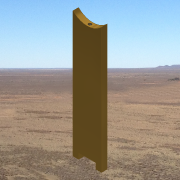
# Autodesk Inventor part: 2f1ar
Saved by Autodesk Inventor 2014 SP1 (Build 180222100, 222)
## iProperties
Company: HERA Project
Created: 2013-12-20
Part Number: 2f1ar
Material: Brass, Soft Yellow
Document SubType Name: Modeling
Designer: Rich Bradley
Mass: 28.2753 g
Surface Area: 26.7824 cm^2
Volume: 3.33829 cm^3
Density: 8.47 g/cm^3
Description: Feed arm pipe rest
Appearance: Brass - Satin
Author: David DeBoer
Title: Dipole Arm Rest
Autodesk Inventor part; units mm, degrees
ref_plane "YZ Plane" through (0, 0, 0) normal (1, 0, 0) x (0, 1, 0)
ref_plane "XZ Plane" through (0, 0, 0) normal (0, 1, 0) x (-1, 0, 0)
sketch "Sketch1" plane through (0, 0, 0) normal (0, 0, 1) x (1, 0, 0)
  line L0 (0, 0) -> (15.875, 0)
  line L1 (15.875, 0) -> (15.875, 77.724)
  line L2 (15.875, 77.724) -> (0, 77.724)
  line L3 (0, 77.724) -> (0, 0)
  dimension "d0" = 77.724
  dimension "d1" = 15.875
  constraints: 8 end point, 2 parallel, 1 horizontal, 1 perpendicular
  measures "d0" distance of L2.end L0.start
  measures "d1" distance of L0.start L0.end
extrude "Extrusion1" add sketch "Sketch1" along normal blind 3.175
sketch "Sketch2" plane through (0, 0, 3.175) normal (0, 0, 1) x (1, 0, 0)
  line L0 (0, 0) -> (15.875, 0) projected
  line L1 (15.875, 77.724) -> (0, 77.724) projected
  line L2 (3.175, 0) -> (12.7, 0)
  line L3 (12.7, 0) -> (12.7, 3.175)
  line L4 (12.7, 3.175) -> (3.175, 3.175)
  line L5 (3.175, 3.175) -> (3.175, 0)
  line L6 (7.9375, 3.175) -> (7.9375, 0) construction
  line L7 (7.9375, 77.724) -> (7.9375, 0) construction
  dimension "d4" = 9.525
  dimension "d6" = 3.175
  constraints: 12 end point, 4 midpoint, 2 collinear, 2 parallel, 1 horizontal, 1 perpendicular
  measures "d4" distance of L3.end L4.end
  measures "d6" distance of L2.end L3.end
extrude "Extrusion2" cut sketch "Sketch2" against normal through all
sketch "Sketch3" plane through (0, 0, 3.175) normal (0, 0, 1) x (1, 0, 0)
  circle A0 centre (7.9375, 77.7875) radius 11.1125
  dimension "d11" = 22.225
  constraints: 1 centre point
  measures "d11" diameter of A0
extrude "Extrusion3" cut sketch "Sketch3" against normal blind 3.175
ref_plane "Work Plane1" through (15.875, 70.0104, 0) normal (0, -1, 0) x (0, 0, 1)
sketch "Sketch6" plane through (15.875, 70.0104, 0) normal (0, -1, 0) x (0, 0, 1)
  line L0 (3.1705, 0.0025) -> (0, 0.0025) construction
  line L1 (1.5853, 0.0025) -> (1.5853, 15.875) construction
  circle A0 centre (1.5853, 7.9388) radius 0.6177
  point P0 (0, 15.875)
  constraints: 4 end point, 2 midpoint, 1 centre point, 1 horizontal, 1 perpendicular
hole "Hole3" at (7.9362, 70.0104, 1.5853) direction (0, -1, 0) diameter 1.7018 depth 33.02 tip angle 118
sketch "Sketch7" plane through (15.875, 0, 0) normal (0, -1, 0) x (1, 0, 0)
  line L0 (-15.875, 0) -> (0, 0) construction
  line L1 (0, 0) -> (0, 3.175) construction
  line L2 (0, 3.175) -> (-15.875, 3.175) construction
  line L3 (-15.875, 3.175) -> (-15.875, 0) construction
  line L4 (-7.9375, 3.175) -> (-7.9375, 0) construction
  circle A0 centre (-14.2875, 1.5875) radius 0.7756
  line L5 (-15.875, 0) -> (-15.875, 3.175) construction
  circle A1 centre (-1.5875, 1.5875) radius 0.7756
  point P0 (-3.175, 3.175)
  dimension "d36" = 15.875
  dimension "d37" = 6.35
  constraints: 12 end point, 2 centre point, 2 midpoint, 2 parallel, 1 horizontal, 1 perpendicular, 1 symmetric about line, 1 other
  measures "d36" distance of L2.end L1.end
  measures "d37" distance from line of A0.centre L4
hole "Hole4" at (14.2875, 0, 1.5875) at (1.5875, 0, 1.5875) direction (0, 1, 0) diameter 1.7018 depth 25.4 tip angle 118
body "Solid1"
